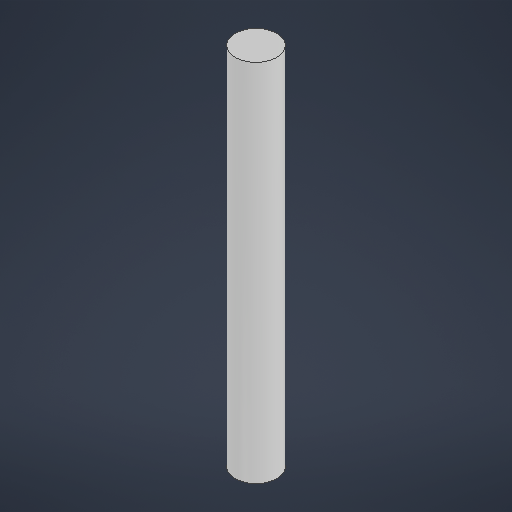
# Autodesk Inventor part: eje8x70mm
Saved by Autodesk Inventor 2026 (Build 300175050, 175E)
## iProperties
Created: 2024-03-11
Part Number: eje8x70mm
Material: Steel
Document SubType Name: Modeling
Designer: diego
Density: 7.85 g/cm^3
Appearance: Aluminum - Polished
Mass: 27.6209 g
Surface Area: 18.5982 cm^2
Volume: 3.51858 cm^3
Author: diego
Autodesk Inventor part; units mm, degrees
ref_plane "YZ Plane" through (0, 0, 0) normal (1, 0, 0) x (0, 1, 0)
ref_plane "XZ Plane" through (0, 0, 0) normal (0, 1, 0) x (-1, 0, 0)
ref_plane "XY Plane" through (0, 0, 0) normal (0, 0, 1) x (1, 0, 0)
sketch "Sketch1" plane through (0, 0, 0) normal (0, 1, 0) x (-1, 0, 0)
  circle A0 centre (0, 0) radius 4
  dimension "d0" = 8
  constraints: 1 centre point, 1 coincident
  measures "d0" diameter of A0
extrude "Extrusion1" add sketch "Sketch1" along normal mid plane 70
body "Solid1"
